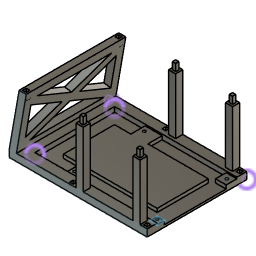
WRO pi EXPANSION BOARD v6 (1) (Autodesk Fusion 360 design; units mm, degrees)
Autodesk Fusion 360 part; units mm, degrees
note: some values were not read from the file. Set by a fixed rule: which sketch regions a step uses.
(part 1 of 2)
sketch "Sketch1" plane through (0, 0, 0) normal (0, 1, 0) x (1, 0, 0)
  line L0 (0, 0) -> (-97, 0)
  line L1 (-97, 0) -> (-97, -5)
  line L2 (-97, -5) -> (0, -5)
  line L3 (0, -5) -> (0, 0)
  dimension "d1" = 97
  dimension "d2" = 5
  constraint horizontal L0
  constraint vertical L1
  constraint horizontal L2
  constraint vertical L3
  constraint coincident L0.start L3.end
  measures "d1" distance of L0.start L0.end
  measures "d2" distance of L0.start L2.end
extrude "Extrude1" add sketch "Sketch1" along normal blind 60
sketch "Sketch2" plane through (0, 0, 5) normal (0, 0, 1) x (-1, 0, 0)
  line L0 (97, 0) -> (0, 0)
  line L1 (0, 0) -> (0, -60)
  line L2 (0, -60) -> (97, -60)
  line L3 (97, -60) -> (97, 0)
  line L4 (0, 0) -> (1.25, 0)
  line L5 (1.25, 0) -> (1.25, -1.25)
  line L6 (1.25, -1.25) -> (3.75, -1.25)
  line L7 (3.75, -1.25) -> (3.75, -3.75)
  line L8 (3.75, -3.75) -> (1.25, -3.75)
  line L9 (1.25, -3.75) -> (1.25, -1.25)
  line L10 (0, -60) -> (0, -58.75)
  line L11 (0, -58.75) -> (1.25, -58.75)
  line L12 (1.25, -58.75) -> (3.75, -58.75)
  line L13 (3.75, -58.75) -> (3.75, -56.25)
  line L14 (3.75, -56.25) -> (1.25, -56.25)
  line L15 (1.25, -56.25) -> (1.25, -58.75)
  line L16 (97, -60) -> (97, -58.75)
  line L17 (97, -58.75) -> (95.75, -58.75)
  line L18 (95.75, -58.75) -> (93.25, -58.75)
  line L19 (93.25, -58.75) -> (93.25, -56.25)
  line L20 (93.25, -56.25) -> (95.75, -56.25)
  line L21 (95.75, -56.25) -> (95.75, -58.75)
  line L22 (97, 0) -> (95.75, 0)
  line L23 (95.75, 0) -> (95.75, -1.25)
  line L24 (95.75, -1.25) -> (93.25, -1.25)
  line L25 (93.25, -1.25) -> (93.25, -3.75)
  line L26 (93.25, -3.75) -> (95.75, -3.75)
  line L27 (95.75, -3.75) -> (95.75, -1.25)
  dimension "d5" = 1.25
  dimension "d6" = 1.25
  dimension "d7" = 2.5
  dimension "d8" = 2.5
  dimension "d9" = 1.25
  dimension "d10" = 1.25
  dimension "d11" = 2.5
  dimension "d12" = 2.5
  dimension "d13" = 1.25
  dimension "d14" = 1.25
  dimension "d15" = 2.5
  dimension "d16" = 2.5
  dimension "d17" = 1.25
  dimension "d18" = 1.25
  dimension "d19" = 2.5
  dimension "d20" = 2.5
  constraint coincident L0.end L1.start
  constraint perpendicular L1 L4
  constraint perpendicular L4 L5
  constraint horizontal L6
  constraint vertical L7
  constraint horizontal L8
  constraint vertical L9
  constraint coincident L1.end L2.start
  constraint perpendicular L2 L10
  constraint perpendicular L10 L11
  constraint horizontal L12
  constraint vertical L13
  constraint horizontal L14
  constraint vertical L15
  constraint coincident L2.end L3.start
  constraint perpendicular L2 L16
  constraint perpendicular L16 L17
  constraint horizontal L18
  constraint vertical L19
  constraint horizontal L20
  constraint vertical L21
  constraint coincident L0.start L3.end
  constraint perpendicular L3 L22
  constraint perpendicular L22 L23
  constraint horizontal L24
  constraint vertical L25
  constraint horizontal L26
  constraint vertical L27
  measures "d5" distance of L0.end L4.end
  measures "d6" distance of L4.end L5.end
  measures "d7" distance of L5.end L6.end
  measures "d8" distance of L5.end L8.end
  measures "d9" distance of L1.end L10.end
  measures "d10" distance of L10.end L11.end
  measures "d11" distance of L11.end L12.end
  measures "d12" distance of L11.end L14.end
  measures "d13" distance of L2.end L16.end
  measures "d14" distance of L16.end L17.end
  measures "d15" distance of L17.end L18.end
  measures "d16" distance of L17.end L20.end
  measures "d17" distance of L0.start L22.end
  measures "d18" distance of L22.end L23.end
  measures "d19" distance of L23.end L24.end
  measures "d20" distance of L23.end L26.end
extrude "Extrude2" cut sketch "Sketch2" against normal blind 1000 contours L6 L7 L8 L9 | L12 L13 L14 L15 | L18 L19 L20 L21 | L24 L25 L26 L27
sketch "Sketch3" plane through (0, 0, 5) normal (0, 0, 1) x (-1, 0, 0)
  line L0 (93.25, -58.75) -> (93.25, -56.25)
  line L1 (93.25, -56.25) -> (95.75, -56.25)
  line L2 (95.75, -56.25) -> (95.75, -58.75)
  line L3 (95.75, -58.75) -> (93.25, -58.75)
  line L4 (3.75, -58.75) -> (1.25, -58.75)
  line L5 (1.25, -58.75) -> (1.25, -56.25)
  line L6 (1.25, -56.25) -> (3.75, -56.25)
  line L7 (3.75, -56.25) -> (3.75, -58.75)
  line L8 (93.25, -1.25) -> (95.75, -1.25)
  line L9 (95.75, -1.25) -> (95.75, -3.75)
  line L10 (95.75, -3.75) -> (93.25, -3.75)
  line L11 (93.25, -3.75) -> (93.25, -1.25)
  line L12 (3.75, -1.25) -> (3.75, -3.75)
  line L13 (3.75, -3.75) -> (1.25, -3.75)
  line L14 (1.25, -3.75) -> (1.25, -1.25)
  line L15 (1.25, -1.25) -> (3.75, -1.25)
  line L16 (97, 0) -> (0, 0)
  line L17 (0, 0) -> (0, -60)
  line L18 (0, -60) -> (97, -60)
  line L19 (97, -60) -> (97, 0)
  line L20 (95.75, -3.75) -> (95.75, -56.25)
  line L21 (95.75, -56.25) -> (95.75, -30)
  line L22 (95.75, -30) -> (95.75, -5)
  line L23 (95.75, -5) -> (95.75, -6.25)
  line L24 (95.75, -6.25) -> (93.25, -6.25)
  line L25 (93.25, -6.25) -> (93.25, -8.75)
  line L26 (93.25, -8.75) -> (95.75, -8.75)
  line L27 (95.75, -8.75) -> (95.75, -6.25)
  line L28 (95.75, -30) -> (95.75, -55)
  line L29 (95.75, -55) -> (95.75, -53.75)
  line L30 (95.75, -53.75) -> (93.25, -53.75)
  line L31 (93.25, -53.75) -> (93.25, -51.25)
  line L32 (93.25, -51.25) -> (95.75, -51.25)
  line L33 (95.75, -51.25) -> (95.75, -53.75)
  line L34 (92, -4) -> (95.75, -4)
  line L35 (95.75, -4) -> (95.75, -0.5684)
  line L36 (95.75, -0.5684) -> (92, -0.5684)
  line L37 (92, -0.5684) -> (92, -4)
  line L38 (93.25, -58.75) -> (96.4667, -58.75)
  line L39 (96.4667, -58.75) -> (96.4667, -55.6639)
  line L40 (96.4667, -55.6639) -> (93.25, -55.6639)
  line L41 (93.25, -55.6639) -> (93.25, -58.75)
  dimension "d23" = 25
  dimension "d24" = 1.25
  dimension "d25" = 2.5
  dimension "d26" = 2.5
  dimension "d27" = 25
  dimension "d28" = 1.25
  dimension "d29" = 2.5
  dimension "d30" = 2.5
  constraint coincident L9.end L10.start
  constraint coincident L1.end L2.start
  constraint midpoint L20 L21.end
  constraint parallel L20 L22
  constraint parallel L20 L23
  constraint horizontal L24
  constraint vertical L25
  constraint horizontal L26
  constraint vertical L27
  constraint parallel L20 L28
  constraint parallel L20 L29
  constraint horizontal L30
  constraint vertical L31
  constraint horizontal L32
  constraint vertical L33
  constraint horizontal L34
  constraint vertical L35
  constraint horizontal L36
  constraint vertical L37
  constraint horizontal L38
  constraint vertical L39
  constraint horizontal L40
  constraint vertical L41
  constraint coincident L0.start L3.end
  measures "d23" distance of L21.end L22.end
  measures "d24" distance of L22.end L23.end
  measures "d25" distance of L23.end L24.end
  measures "d26" distance of L23.end L26.end
  measures "d27" distance of L21.end L28.end
  measures "d28" distance of L28.end L29.end
  measures "d29" distance of L29.end L30.end
  measures "d30" distance of L29.end L32.end
extrude "Extrude3" cut sketch "Sketch3" against normal blind 5 contours L0 L1 L2 L3 L38 L41 | L8 L9 L10 L11 L35 | L20 L22 L24 L25 L26 L27 | L20 L21 L28 L30 L31 L32 L33
sketch "Sketch4" plane through (0, 0, 5) normal (0, 0, 1) x (-1, 0, 0)
  line L0 (93.25, -6.25) -> (95.75, -6.25)
  line L1 (95.75, -6.25) -> (95.75, -8.75)
  line L2 (95.75, -8.75) -> (93.25, -8.75)
  line L3 (93.25, -8.75) -> (93.25, -6.25)
  line L4 (93.25, -53.75) -> (93.25, -51.25)
  line L5 (93.25, -51.25) -> (95.75, -51.25)
  line L6 (95.75, -51.25) -> (95.75, -53.75)
  line L7 (95.75, -53.75) -> (93.25, -53.75)
  line L8 (93.25, -58.75) -> (93.25, -56.25)
  line L9 (93.25, -56.25) -> (95.75, -56.25)
  line L10 (95.75, -56.25) -> (95.75, -58.75)
  line L11 (95.75, -58.75) -> (93.25, -58.75)
  line L12 (3.75, -58.75) -> (1.25, -58.75)
  line L13 (1.25, -58.75) -> (1.25, -56.25)
  line L14 (1.25, -56.25) -> (3.75, -56.25)
  line L15 (3.75, -56.25) -> (3.75, -58.75)
  line L16 (93.25, -1.25) -> (95.75, -1.25)
  line L17 (95.75, -1.25) -> (95.75, -3.75)
  line L18 (95.75, -3.75) -> (93.25, -3.75)
  line L19 (93.25, -3.75) -> (93.25, -1.25)
  line L20 (3.75, -1.25) -> (3.75, -3.75)
  line L21 (3.75, -3.75) -> (1.25, -3.75)
  line L22 (1.25, -3.75) -> (1.25, -1.25)
  line L23 (1.25, -1.25) -> (3.75, -1.25)
  line L24 (97, 0) -> (0, 0)
  line L25 (0, 0) -> (0, -60)
  line L26 (0, -60) -> (97, -60)
  line L27 (97, -60) -> (97, 0)
  line L28 (91.453, -0.7924) -> (95.75, -0.7924)
  line L29 (95.75, -0.7924) -> (95.75, -4.5214)
  line L30 (95.75, -4.5214) -> (91.453, -4.5214)
  line L31 (91.453, -4.5214) -> (91.453, -0.7924)
  line L32 (91.453, -55.7947) -> (95.75, -55.7947)
  line L33 (95.75, -55.7947) -> (95.75, -59.4305)
  line L34 (95.75, -59.4305) -> (91.453, -59.4305)
  line L35 (91.453, -59.4305) -> (91.453, -55.7947)
  constraint horizontal L28
  constraint vertical L29
  constraint horizontal L30
  constraint vertical L31
  constraint horizontal L32
  constraint vertical L33
  constraint horizontal L34
  constraint vertical L35
extrude "Extrude4" add sketch "Sketch4" against normal blind 5 contours L8 L9 L10 L11 L33 | L16 L17 L18 L19 L29
extrude "Extrude5" add 1 faces at (-64.6667, 60, 1.6667) along direction (0, 1, 0) blind 5
extrude "Extrude6" add 1 faces at (-64.6667, 0, 1.6667) along direction (0, -1, 0) blind 5
sketch "Sketch5" plane through (0, 0, 5) normal (0, 0, 1) x (-1, 0, 0)
  line L0 (93.25, -6.25) -> (95.75, -6.25)
  line L1 (95.75, -6.25) -> (95.75, -8.75)
  line L2 (95.75, -8.75) -> (93.25, -8.75)
  line L3 (93.25, -8.75) -> (93.25, -6.25)
  line L4 (93.25, -53.75) -> (93.25, -51.25)
  line L5 (93.25, -51.25) -> (95.75, -51.25)
  line L6 (95.75, -51.25) -> (95.75, -53.75)
  line L7 (95.75, -53.75) -> (93.25, -53.75)
  line L8 (3.75, -58.75) -> (1.25, -58.75)
  line L9 (1.25, -58.75) -> (1.25, -56.25)
  line L10 (1.25, -56.25) -> (3.75, -56.25)
  line L11 (3.75, -56.25) -> (3.75, -58.75)
  line L12 (3.75, -1.25) -> (3.75, -3.75)
  line L13 (3.75, -3.75) -> (1.25, -3.75)
  line L14 (1.25, -3.75) -> (1.25, -1.25)
  line L15 (1.25, -1.25) -> (3.75, -1.25)
  line L16 (0, 5) -> (0, -65)
  line L17 (0, -65) -> (97, -65)
  line L18 (97, -65) -> (97, 5)
  line L19 (97, 5) -> (0, 5)
  line L20 (1.25, -1.25) -> (1.25, 3.75)
  line L21 (1.25, 3.75) -> (3.75, 3.75)
  line L22 (3.75, 3.75) -> (3.75, 1.25)
  line L23 (3.75, 1.25) -> (1.25, 1.25)
  line L24 (1.25, 1.25) -> (1.25, 3.75)
  line L25 (1.25, -58.75) -> (1.25, -63.75)
  line L26 (1.25, -63.75) -> (3.75, -63.75)
  line L27 (3.75, -63.75) -> (3.75, -61.25)
  line L28 (3.75, -61.25) -> (1.25, -61.25)
  line L29 (1.25, -61.25) -> (1.25, -63.75)
  dimension "d39" = 5
  dimension "d40" = 2.5
  dimension "d41" = 2.5
  dimension "d42" = 5
  dimension "d43" = 2.5
  dimension "d44" = 2.5
  constraint coincident L14.end L15.start
  constraint perpendicular L15 L20
  constraint horizontal L21
  constraint vertical L22
  constraint horizontal L23
  constraint vertical L24
  constraint coincident L8.end L9.start
  constraint perpendicular L8 L25
  constraint horizontal L26
  constraint vertical L27
  constraint horizontal L28
  constraint vertical L29
  measures "d39" distance of L14.end L20.end
  measures "d40" distance of L20.end L21.end
  measures "d41" distance of L20.end L23.end
  measures "d42" distance of L8.end L25.end
  measures "d43" distance of L25.end L26.end
  measures "d44" distance of L25.end L28.end
extrude "Extrude7" cut sketch "Sketch5" against normal blind 5000 contours L20 L21 L22 L23 L24 | L25 L26 L27 L28 L29
sketch "Sketch6" plane through (0, 0, 5) normal (0, 0, 1) x (-1, 0, 0)
  line L0 (3.75, 3.75) -> (3.75, 1.25)
  line L1 (3.75, 1.25) -> (1.25, 1.25)
  line L2 (1.25, 1.25) -> (1.25, 3.75)
  line L3 (1.25, 3.75) -> (3.75, 3.75)
  line L4 (3.75, -63.75) -> (1.25, -63.75)
  line L5 (1.25, -63.75) -> (1.25, -61.25)
  line L6 (1.25, -61.25) -> (3.75, -61.25)
  line L7 (3.75, -61.25) -> (3.75, -63.75)
  line L8 (93.25, -6.25) -> (95.75, -6.25)
  line L9 (95.75, -6.25) -> (95.75, -8.75)
  line L10 (95.75, -8.75) -> (93.25, -8.75)
  line L11 (93.25, -8.75) -> (93.25, -6.25)
  line L12 (93.25, -53.75) -> (93.25, -51.25)
  line L13 (93.25, -51.25) -> (95.75, -51.25)
  line L14 (95.75, -51.25) -> (95.75, -53.75)
  line L15 (95.75, -53.75) -> (93.25, -53.75)
  line L16 (3.75, -58.75) -> (1.25, -58.75)
  line L17 (1.25, -58.75) -> (1.25, -56.25)
  line L18 (1.25, -56.25) -> (3.75, -56.25)
  line L19 (3.75, -56.25) -> (3.75, -58.75)
  line L20 (3.75, -1.25) -> (3.75, -3.75)
  line L21 (3.75, -3.75) -> (1.25, -3.75)
  line L22 (1.25, -3.75) -> (1.25, -1.25)
  line L23 (1.25, -1.25) -> (3.75, -1.25)
  line L24 (0, 5) -> (0, -65)
  line L25 (0, -65) -> (97, -65)
  line L26 (97, -65) -> (97, 5)
  line L27 (97, 5) -> (0, 5)
  line L28 (1.25, -58.75) -> (10, -58.75)
  line L29 (10, -58.75) -> (10, 0)
  line L30 (10, 0) -> (1.25, 0)
  line L31 (1.25, 0) -> (1.25, -58.75)
  constraint horizontal L28
  constraint vertical L29
  constraint horizontal L30
  constraint vertical L31
  constraint coincident L16.end L17.start
extrude "Extrude8" add sketch "Sketch6" against normal blind 5 contours L16 L17 L18 L19 L28 L31 | L20 L21 L22 L23 L31
sketch "Sketch7" plane through (0, 0, 5) normal (0, 0, 1) x (-1, 0, 0)
  line L0 (3.75, 3.75) -> (3.75, 1.25)
  line L1 (3.75, 1.25) -> (1.25, 1.25)
  line L2 (1.25, 1.25) -> (1.25, 3.75)
  line L3 (1.25, 3.75) -> (3.75, 3.75)
  line L4 (3.75, -63.75) -> (1.25, -63.75)
  line L5 (1.25, -63.75) -> (1.25, -61.25)
  line L6 (1.25, -61.25) -> (3.75, -61.25)
  line L7 (3.75, -61.25) -> (3.75, -63.75)
  line L8 (93.25, -6.25) -> (95.75, -6.25)
  line L9 (95.75, -6.25) -> (95.75, -8.75)
  line L10 (95.75, -8.75) -> (93.25, -8.75)
  line L11 (93.25, -8.75) -> (93.25, -6.25)
  line L12 (93.25, -53.75) -> (93.25, -51.25)
  line L13 (93.25, -51.25) -> (95.75, -51.25)
  line L14 (95.75, -51.25) -> (95.75, -53.75)
  line L15 (95.75, -53.75) -> (93.25, -53.75)
  line L16 (0, 5) -> (0, -65)
  line L17 (0, -65) -> (97, -65)
  line L18 (97, -65) -> (97, 5)
  line L19 (97, 5) -> (0, 5)
  line L20 (3.75, 3.75) -> (53.25, 3.75)
  line L21 (53.25, 3.75) -> (55.75, 3.75)
  line L22 (55.75, 3.75) -> (55.75, 1.25)
  line L23 (55.75, 1.25) -> (53.25, 1.25)
  line L24 (53.25, 1.25) -> (53.25, 3.75)
  line L25 (3.75, -63.75) -> (53.25, -63.75)
  line L26 (53.25, -63.75) -> (55.75, -63.75)
  line L27 (55.75, -63.75) -> (55.75, -61.25)
  line L28 (55.75, -61.25) -> (53.25, -61.25)
  line L29 (53.25, -61.25) -> (53.25, -63.75)
  dimension "d49" = 49.5
  dimension "d50" = 2.5
  dimension "d51" = 2.5
  dimension "d52" = 49.5
  dimension "d53" = 2.5
  dimension "d54" = 2.5
  constraint coincident L0.start L3.end
  constraint perpendicular L0 L20
  constraint horizontal L21
  constraint vertical L22
  constraint horizontal L23
  constraint vertical L24
  constraint coincident L4.start L7.end
  constraint perpendicular L7 L25
  constraint horizontal L26
  constraint vertical L27
  constraint horizontal L28
  constraint vertical L29
  measures "d49" distance of L0.start L20.end
  measures "d50" distance of L20.end L21.end
  measures "d51" distance of L20.end L23.end
  measures "d52" distance of L4.start L25.end
  measures "d53" distance of L25.end L26.end
  measures "d54" distance of L25.end L28.end
extrude "Extrude9" cut sketch "Sketch7" against normal blind 150 contours L21 L22 L23 L24 | L26 L27 L28 L29
sketch "Sketch8" plane through (0, 0, 5) normal (0, 0, 1) x (-1, 0, 0)
  line L0 (55.75, 3.75) -> (55.75, 1.25)
  line L1 (55.75, 1.25) -> (53.25, 1.25)
  line L2 (53.25, 1.25) -> (53.25, 3.75)
  line L3 (53.25, 3.75) -> (55.75, 3.75)
  line L4 (55.75, -63.75) -> (53.25, -63.75)
  line L5 (53.25, -63.75) -> (53.25, -61.25)
  line L6 (53.25, -61.25) -> (55.75, -61.25)
  line L7 (55.75, -61.25) -> (55.75, -63.75)
  line L8 (3.75, 3.75) -> (3.75, 1.25)
  line L9 (3.75, 1.25) -> (1.25, 1.25)
  line L10 (1.25, 1.25) -> (1.25, 3.75)
  line L11 (1.25, 3.75) -> (3.75, 3.75)
  line L12 (3.75, -63.75) -> (1.25, -63.75)
  line L13 (1.25, -63.75) -> (1.25, -61.25)
  line L14 (1.25, -61.25) -> (3.75, -61.25)
  line L15 (3.75, -61.25) -> (3.75, -63.75)
  line L16 (93.25, -6.25) -> (95.75, -6.25)
  line L17 (95.75, -6.25) -> (95.75, -8.75)
  line L18 (95.75, -8.75) -> (93.25, -8.75)
  line L19 (93.25, -8.75) -> (93.25, -6.25)
  line L20 (93.25, -53.75) -> (93.25, -51.25)
  line L21 (93.25, -51.25) -> (95.75, -51.25)
  line L22 (95.75, -51.25) -> (95.75, -53.75)
  line L23 (95.75, -53.75) -> (93.25, -53.75)
  line L24 (0, 5) -> (0, -65)
  line L25 (0, -65) -> (97, -65)
  line L26 (97, -65) -> (97, 5)
  line L27 (97, 5) -> (0, 5)
  line L28 (86.4798, -65) -> (86.4798, -30)
  line L29 (86.4798, -30) -> (86.4798, -2)
  line L30 (86.4798, -2) -> (0.4798, -2)
  line L31 (0.4798, -2) -> (0.4798, -58)
  line L32 (0.4798, -58) -> (86.4798, -58)
  line L33 (86.4798, -58) -> (86.4798, -2)
  dimension "d57" = 35
  dimension "d58" = 28
  dimension "d59" = 86
  dimension "d60" = 56
  constraint coincident L25 L28.start
  constraint perpendicular L27 L28
  constraint perpendicular L25 L29
  constraint horizontal L30
  constraint vertical L31
  constraint horizontal L32
  constraint vertical L33
  measures "d57" distance of L28.start L28.end
  measures "d58" distance of L28.end L29.end
  measures "d59" distance of L29.end L30.end
  measures "d60" distance of L29.end L32.end
extrude "Extrude10" cut sketch "Sketch8" against normal blind 1 contours L28 L29 L30 L31 L32 L33
sketch "Sketch9" plane through (0, 0, 5) normal (0, 0, 1) x (-1, 0, 0)
  line L0 (0.4798, -2) -> (86.4798, -2)
  line L1 (86.4798, -2) -> (86.4798, -58)
  line L2 (86.4798, -58) -> (0.4798, -58)
  line L3 (0.4798, -58) -> (0.4798, -2)
  line L4 (55.75, 3.75) -> (55.75, 1.25)
  line L5 (55.75, 1.25) -> (53.25, 1.25)
  line L6 (53.25, 1.25) -> (53.25, 3.75)
  line L7 (53.25, 3.75) -> (55.75, 3.75)
  line L8 (55.75, -63.75) -> (53.25, -63.75)
  line L9 (53.25, -63.75) -> (53.25, -61.25)
  line L10 (53.25, -61.25) -> (55.75, -61.25)
  line L11 (55.75, -61.25) -> (55.75, -63.75)
  line L12 (3.75, 3.75) -> (3.75, 1.25)
  line L13 (3.75, 1.25) -> (1.25, 1.25)
  line L14 (1.25, 1.25) -> (1.25, 3.75)
  line L15 (1.25, 3.75) -> (3.75, 3.75)
  line L16 (3.75, -63.75) -> (1.25, -63.75)
  line L17 (1.25, -63.75) -> (1.25, -61.25)
  line L18 (1.25, -61.25) -> (3.75, -61.25)
  line L19 (3.75, -61.25) -> (3.75, -63.75)
  line L20 (93.25, -6.25) -> (95.75, -6.25)
  line L21 (95.75, -6.25) -> (95.75, -8.75)
  line L22 (95.75, -8.75) -> (93.25, -8.75)
  line L23 (93.25, -8.75) -> (93.25, -6.25)
  line L24 (93.25, -53.75) -> (93.25, -51.25)
  line L25 (93.25, -51.25) -> (95.75, -51.25)
  line L26 (95.75, -51.25) -> (95.75, -53.75)
  line L27 (95.75, -53.75) -> (93.25, -53.75)
  line L28 (0, 5) -> (0, -65)
  line L29 (0, -65) -> (97, -65)
  line L30 (97, -65) -> (97, 5)
  line L31 (97, 5) -> (0, 5)
  line L32 (86.4798, -2) -> (85.9998, -2)
  line L33 (85.9998, -2) -> (85.9998, -59.3993)
  line L34 (85.9998, -59.3993) -> (86.4798, -59.3993)
  line L35 (86.4798, -59.3993) -> (86.4798, -2)
  dimension "d63" = 0.48
  constraint horizontal L32
  constraint vertical L33
  constraint horizontal L34
  constraint vertical L35
  constraint coincident L0.end L1.start
  measures "d63" distance of L0.end L32.end
extrude "Extrude11" add sketch "Sketch9" against normal blind 2 contours L0 L1 L2 L32 L33 L35
sketch "Sketch10" plane through (0, 0, 5) normal (0, 0, 1) x (-1, 0, 0)
  line L0 (0.4798, -2) -> (85.9998, -2)
  line L1 (85.9998, -2) -> (85.9998, -58)
  line L2 (85.9998, -58) -> (0.4798, -58)
  line L3 (0.4798, -58) -> (0.4798, -2)
  line L4 (55.75, 3.75) -> (55.75, 1.25)
  line L5 (55.75, 1.25) -> (53.25, 1.25)
  line L6 (53.25, 1.25) -> (53.25, 3.75)
  line L7 (53.25, 3.75) -> (55.75, 3.75)
  line L8 (55.75, -63.75) -> (53.25, -63.75)
  line L9 (53.25, -63.75) -> (53.25, -61.25)
  line L10 (53.25, -61.25) -> (55.75, -61.25)
  line L11 (55.75, -61.25) -> (55.75, -63.75)
  line L12 (3.75, 3.75) -> (3.75, 1.25)
  line L13 (3.75, 1.25) -> (1.25, 1.25)
  line L14 (1.25, 1.25) -> (1.25, 3.75)
  line L15 (1.25, 3.75) -> (3.75, 3.75)
  line L16 (3.75, -63.75) -> (1.25, -63.75)
  line L17 (1.25, -63.75) -> (1.25, -61.25)
  line L18 (1.25, -61.25) -> (3.75, -61.25)
  line L19 (3.75, -61.25) -> (3.75, -63.75)
  line L20 (93.25, -6.25) -> (95.75, -6.25)
  line L21 (95.75, -6.25) -> (95.75, -8.75)
  line L22 (95.75, -8.75) -> (93.25, -8.75)
  line L23 (93.25, -8.75) -> (93.25, -6.25)
  line L24 (93.25, -53.75) -> (93.25, -51.25)
  line L25 (93.25, -51.25) -> (95.75, -51.25)
  line L26 (95.75, -51.25) -> (95.75, -53.75)
  line L27 (95.75, -53.75) -> (93.25, -53.75)
  line L28 (0, 5) -> (0, -65)
  line L29 (0, -65) -> (97, -65)
  line L30 (97, -65) -> (97, 5)
  line L31 (97, 5) -> (0, 5)
  line L32 (0.4798, -58) -> (-1.0163, -58)
  line L33 (-1.0163, -58) -> (-1.0163, -2)
  line L34 (-1.0163, -2) -> (0.4798, -2)
  line L35 (0.4798, -2) -> (0.4798, -58)
  constraint horizontal L32
  constraint vertical L33
  constraint horizontal L34
  constraint vertical L35
  constraint coincident L2.end L3.start
extrude "Extrude12" cut sketch "Sketch10" against normal blind 1 contours L3 L28 L32 L34 L35
sketch "Sketch11" plane through (0, 0, 4) normal (0, 0, 1) x (-1, 0, 0)
  line L0 (85.9998, -58) -> (85.9998, -2)
  line L1 (85.9998, -2) -> (0, -2)
  line L2 (0, -2) -> (0, -58)
  line L3 (0, -58) -> (85.9998, -58)
  line L4 (0, -58) -> (2.5, -58)
  line L5 (2.5, -58) -> (2.5, -55.5)
  line L6 (2.5, -55.5) -> (3.5, -55.5)
  line L7 (3.5, -55.5) -> (3.5, -54.5)
  circle A0 centre (3.5, -54.5) radius 1
  line L8 (0, -2) -> (3.5, -2)
  line L9 (3.5, -2) -> (3.5, -5.5)
  circle A1 centre (3.5, -5.5) radius 1
  dimension "d68" = 2.5
  dimension "d69" = 2.5
  dimension "d70" = 1
  dimension "d71" = 1
  dimension "d72" = 2
  dimension "d73" = 3.5
  dimension "d74" = 3.5
  dimension "d75" = 2
  constraint coincident L2.end L3.start
  constraint perpendicular L2 L4
  constraint perpendicular L4 L5
  constraint perpendicular L5 L6
  constraint perpendicular L6 L7
  constraint coincident L7.end A0.centre
  constraint coincident L1.end L2.start
  constraint perpendicular L2 L8
  constraint perpendicular L8 L9
  constraint coincident L9.end A1.centre
  measures "d68" distance of L2.end L4.end
  measures "d69" distance of L4.end L5.end
  measures "d70" distance of L5.end L6.end
  measures "d71" distance of L6.end L7.end
  measures "d72" diameter of A0
  measures "d73" distance of L1.end L8.end
  measures "d74" distance of L8.end L9.end
  measures "d75" diameter of A1
extrude "Extrude13" cut sketch "Sketch11" against normal blind 100 contours A0 | A1
sketch "Sketch12" plane through (0, 0, 4) normal (0, 0, 1) x (-1, 0, 0)
  circle A0 centre (3.5, -5.5) radius 1
  circle A1 centre (3.5, -54.5) radius 1
  line L0 (85.9998, -58) -> (85.9998, -2)
  line L1 (5, -7) -> (0, -7)
  line L2 (0, -7) -> (0, -2)
  line L3 (0, -2) -> (5, -2)
  line L4 (5, -2) -> (5, -7)
  constraint horizontal L1
  constraint vertical L2
  constraint horizontal L3
  constraint vertical L4
sketch "Sketch13" plane through (0, 0, 4) normal (0, 0, 1) x (-1, 0, 0)
sketch "Sketch14" plane through (0, 0, 4) normal (0, 0, 1) x (-1, 0, 0)
  line L0 (0, -58) -> (3.5, -58)
  line L1 (3.5, -58) -> (3.5, -54.5)
  line L2 (3.5, -54.5) -> (61.5, -54.5)
  circle A0 centre (61.5, -54.5) radius 1
  line L3 (61.5, -54.5) -> (61.5, -5.5)
  circle A1 centre (61.5, -5.5) radius 1
  dimension "d82" = 3.5
  dimension "d83" = 3.5
  dimension "d84" = 58
  dimension "d85" = 2
  dimension "d86" = 49
  dimension "d87" = 2
  constraint horizontal L0
  constraint perpendicular L0 L1
  constraint perpendicular L1 L2
  constraint coincident L2.end A0.centre
  constraint perpendicular L2 L3
  constraint coincident L3.end A1.centre
  measures "d82" distance of L0.start L0.end
  measures "d83" distance of L0.end L1.end
  measures "d84" distance of L1.end L2.end
  measures "d85" diameter of A0
  measures "d86" distance of L2.end L3.end
  measures "d87" diameter of A1
extrude "Extrude14" cut sketch "Sketch14" against normal blind 500
sketch "Sketch15" plane through (0, 0, 4) normal (0, 0, 1) x (-1, 0, 0)
  circle A0 centre (61.5, -54.5) radius 1
  circle A1 centre (61.5, -5.5) radius 1
  circle A2 centre (3.5, -5.5) radius 1
  circle A3 centre (3.5, -54.5) radius 1
  line L0 (85.9998, -58) -> (85.9998, -2)
  line L1 (85.9998, -2) -> (0, -2)
  line L2 (0, -2) -> (0, -58)
  line L3 (0, -58) -> (85.9998, -58)
  line L4 (0, -58) -> (0, -2)
  line L5 (64.5, -58) -> (52.5, -58)
  line L6 (52.5, -58) -> (52.5, -51)
  line L7 (64.5, -51) -> (64.5, -58)
  line L8 (60.5, -5.5) -> (57.5, -5.5)
  line L9 (62.5, -5.5) -> (64, -5.5)
  line L10 (57.5, -5.5) -> (57.5, -2)
  line L11 (57.5, -2) -> (64, -2)
  line L12 (64, -2) -> (64, -9)
  line L13 (57.5, -9) -> (57.5, -2)
  line L14 (64.5, -58) -> (52.5, -58)
  line L15 (52.5, -58) -> (52.5, -48)
  line L16 (52.5, -48) -> (64.5, -48)
  line L17 (64.5, -48) -> (64.5, -58)
  line L18 (57.5, -2) -> (64, -2)
  line L19 (64, -2) -> (64, -12)
  line L20 (64, -12) -> (57.5, -12)
  line L21 (57.5, -12) -> (57.5, -2)
  line L22 (0, -43) -> (10, -43)
  line L23 (10, -43) -> (10, -58)
  line L24 (52.5, -48) -> (10, -48)
  line L25 (64, -12) -> (76, -12)
  line L26 (76, -12) -> (10, -12)
  line L27 (10, -12) -> (10, -48)
  line L28 (10, -48) -> (76, -48)
  line L29 (76, -48) -> (76, -12)
  dimension "d92" = 7
  dimension "d93" = 3
  dimension "d94" = 1.5
  dimension "d95" = 7
  dimension "d96" = 10
  dimension "d97" = 10
  dimension "d98" = 10
  dimension "d99" = 12
  constraint coincident L2.end L3.start
  constraint coincident L1.end L2.start
  constraint horizontal L5
  constraint vertical L6
  constraint vertical L7
  constraint coincident L3 L5.start
  constraint coincident A1 L8.start
  constraint parallel L1 L8
  constraint coincident A1 L9.start
  constraint parallel L1 L9
  constraint coincident L1 L10.end
  constraint perpendicular L1 L10
  constraint horizontal L11
  constraint vertical L12
  constraint vertical L13
  constraint horizontal L14
  constraint vertical L15
  constraint horizontal L16
  constraint vertical L17
  constraint horizontal L18
  constraint vertical L19
  constraint horizontal L20
  constraint vertical L21
  constraint coincident L4 L22.start
  constraint perpendicular L4 L22
  constraint coincident L3 L23.end
  constraint perpendicular L3 L23
  constraint coincident L23 L24.end
  constraint perpendicular L23 L24
  constraint perpendicular L0 L25
  constraint horizontal L26
  constraint vertical L27
  constraint horizontal L28
  constraint vertical L29
  measures "d92" distance of L5.start L7.start
  measures "d93" distance of L8.start L8.end
  measures "d94" distance of L9.start L9.end
  measures "d95" distance of L10.end L13.start
  measures "d96" distance of L5.start L16.end
  measures "d97" distance of L10.end L20.end
  measures "d98" distance of L22.start L22.end
  measures "d99" distance of L19.end L25.end
extrude "Extrude15" cut sketch "Sketch15" against normal blind 2.5 contours L0 L1 L3 L7 L12 L17 L19 L25 L26 L28 L29 | L3 L6 L15 L23 L24 L28
sketch "Sketch16" plane through (0, 0, 4) normal (0, 0, 1) x (-1, 0, 0)
  circle A0 centre (3.5, -54.5) radius 1
  circle A1 centre (3.5, -5.5) radius 1
  circle A2 centre (61.5, -5.5) radius 1
  circle A3 centre (61.5, -54.5) radius 1
  line L0 (10, -58) -> (10, -48)
  line L1 (10, -48) -> (52.5, -48)
  line L2 (52.5, -48) -> (52.5, -58)
  line L3 (52.5, -58) -> (64.5, -58)
  line L4 (64.5, -58) -> (64.5, -48)
  line L5 (64.5, -48) -> (76, -48)
  line L6 (76, -48) -> (76, -12)
  line L7 (76, -12) -> (64, -12)
  line L8 (64, -12) -> (64, -2)
  line L9 (64, -2) -> (0, -2)
  line L10 (0, -2) -> (0, -58)
  line L11 (0, -58) -> (10, -58)
  line L12 (0, -58) -> (7.5, -58)
  line L13 (7.5, -58) -> (7.5, -50.5)
  line L14 (7.5, -50.5) -> (0, -50.5)
  line L15 (0, -50.5) -> (0, -58)
  line L16 (0, -2) -> (5, -2)
  line L17 (5, -2) -> (5, -7)
  line L18 (5, -7) -> (0, -7)
  line L19 (0, -7) -> (0, -2)
  line L20 (10, -48) -> (76, -48)
  line L21 (76, -48) -> (76, -12)
  line L22 (76, -12) -> (10, -12)
  line L23 (10, -12) -> (10, -48)
  line L24 (64, -2) -> (57.5, -2)
  line L25 (57.5, -2) -> (57.5, -13.1348)
  line L26 (57.5, -13.1348) -> (64, -13.1348)
  line L27 (64, -13.1348) -> (64, -2)
  dimension "d102" = 7.5
  dimension "d103" = 7.5
  dimension "d104" = 6.5
  constraint horizontal L12
  constraint vertical L13
  constraint horizontal L14
  constraint vertical L15
  constraint coincident L10.end L11.start
  constraint horizontal L16
  constraint vertical L17
  constraint horizontal L18
  constraint vertical L19
  constraint coincident L9.end L10.start
  constraint horizontal L20
  constraint vertical L21
  constraint horizontal L22
  constraint vertical L23
  constraint coincident L6.end L7.start
  constraint coincident L0.end L1.start
  constraint horizontal L24
  constraint vertical L25
  constraint horizontal L26
  constraint vertical L27
  constraint coincident L8.end L9.start
  measures "d102" distance of L10.end L12.end
  measures "d103" distance of L10.end L14.end
  measures "d104" distance of L8.end L24.end
extrude "Extrude16" cut sketch "Sketch16" against normal blind 2.5 contours L0 L9 L10 L11 L13 L14 L17 L18 L22 L23 L25
sketch "Sketch17" plane through (0, -5, 0) normal (0, -1, 0) x (1, 0, 0)
  line L0 (0, 0) -> (0, 5)
  line L1 (0, 5) -> (-97, 5)
  line L2 (-97, 5) -> (-97, 0)
  line L3 (-97, 0) -> (0, 0)
  line L4 (-97, 5) -> (-90.0541, 44.3923)
  line L5 (-97, 5) -> (-57, 5) construction
  line L6 (-92.3722, 31.2455) -> (-87.6738, 29.5354)
  line L7 (-92.3722, 31.2455) -> (-87.3722, 31.2455) construction
  line L8 (-94.8047, 17.45) -> (-90.1063, 15.7399)
  line L9 (-94.8047, 17.45) -> (-89.8047, 17.45) construction
  line L10 (-87.6738, 29.5354) -> (-92, 5)
  line L11 (-87.6738, 29.5354) -> (-62.7599, 29.5354) construction
  line L12 (-92, 5) -> (-85.0541, 44.3923)
  line L13 (-90.0541, 44.3923) -> (-85.0541, 44.3923)
  dimension "d107" = 80
  dimension "d108" = 40
  dimension "d109" = 20
  dimension "d110" = 5
  dimension "d111" = 20
  dimension "d112" = 5
  dimension "d113" = 100
  dimension "d114" = 40
  constraint horizontal L5
  constraint coincident L1.end L2.start
  constraint horizontal L7
  constraint coincident L4 L6.start
  constraint horizontal L9
  constraint coincident L4 L8.start
  constraint horizontal L11
  constraint coincident L5 L10.end
  constraint parallel L10 L12
  measures "d107" angle of L4 L5
  measures "d108" distance of L1.end L4.end
  measures "d109" angle of L6 L7
  measures "d110" distance of L6.start L6.end
  measures "d111" angle of L8 L9
  measures "d112" distance of L8.start L8.end
  measures "d113" angle of L10 L11
  measures "d114" distance of L10.end L12.end
extrude "Extrude17" add sketch "Sketch17" against normal blind 70 contours L1 L4 L8 L10 L12 | L4 L6 L8 L10 L12 | L4 L6 L12 L13
sketch "Sketch18" plane through (0, -5, 0) normal (0, -1, 0) x (1, 0, 0)
  line L0 (0, 0) -> (0, 5)
  line L1 (0, 5) -> (-92, 5)
  line L2 (-92, 5) -> (-85.0541, 44.3923)
  line L3 (-85.0541, 44.3923) -> (-90.0541, 44.3923)
  line L4 (-90.0541, 44.3923) -> (-97, 5)
  line L5 (-97, 5) -> (-97, 0)
  line L6 (-97, 0) -> (0, 0)
sketch "Sketch19" plane through (0, 0, 44.3923) normal (0, 0, 1) x (-1, 0, 0)
  line L0 (90.0541, 5) -> (85.0541, 5)
  line L1 (85.0541, 5) -> (85.0541, -65)
  line L2 (85.0541, -65) -> (90.0541, -65)
  line L3 (90.0541, -65) -> (90.0541, 5)
  line L4 (90.0541, 5) -> (90.0541, 3.65)
  line L5 (90.0541, 3.65) -> (88.7041, 3.65)
  line L6 (88.7041, 3.65) -> (86.4041, 3.65)
  line L7 (86.4041, 3.65) -> (86.4041, 1.35)
  line L8 (86.4041, 1.35) -> (88.7041, 1.35)
  line L9 (88.7041, 1.35) -> (88.7041, 3.65)
  dimension "d117" = 1.35
  dimension "d118" = 1.35
  dimension "d119" = 2.3
  dimension "d120" = 2.3
  constraint coincident L0.start L3.end
  constraint perpendicular L0 L4
  constraint perpendicular L4 L5
  constraint horizontal L6
  constraint vertical L7
  constraint horizontal L8
  constraint vertical L9
  measures "d117" distance of L0.start L4.end
  measures "d118" distance of L4.end L5.end
  measures "d119" distance of L5.end L6.end
  measures "d120" distance of L5.end L8.end
extrude "Extrude18" add sketch "Sketch19" along normal blind 5 contours L6 L7 L8 L9
sketch "Sketch20" plane through (0, 0, 44.3923) normal (0, 0, 1) x (-1, 0, 0)
  line L0 (88.7041, 1.35) -> (86.4041, 1.35)
  line L1 (86.4041, 1.35) -> (86.4041, 3.65)
  line L2 (86.4041, 3.65) -> (88.7041, 3.65)
  line L3 (88.7041, 3.65) -> (88.7041, 1.35)
  line L4 (90.0541, 5) -> (85.0541, 5)
  line L5 (85.0541, 5) -> (85.0541, -65)
  line L6 (85.0541, -65) -> (90.0541, -65)
  line L7 (90.0541, -65) -> (90.0541, 5)
  line L8 (90.0541, -65) -> (88.8041, -65)
  line L9 (88.8041, -65) -> (88.8041, -63.75)
  line L10 (88.8041, -63.75) -> (90.0541, -63.75)
  line L11 (90.0541, -63.75) -> (90.0541, -65)
  line L12 (88.8041, -63.75) -> (86.5041, -63.75)
  line L13 (86.5041, -63.75) -> (86.5041, -61.45)
  line L14 (86.5041, -61.45) -> (88.8041, -61.45)
  line L15 (88.8041, -61.45) -> (88.8041, -63.75)
  dimension "d123" = 1.25
  dimension "d124" = 1.25
  dimension "d125" = 2.3
  dimension "d126" = 2.3
  constraint horizontal L8
  constraint vertical L9
  constraint horizontal L10
  constraint vertical L11
  constraint coincident L6.end L7.start
  constraint horizontal L12
  constraint vertical L13
  constraint horizontal L14
  constraint vertical L15
  measures "d123" distance of L6.end L8.end
  measures "d124" distance of L6.end L10.end
  measures "d125" distance of L9.end L12.end
  measures "d126" distance of L9.end L14.end
extrude "Extrude19" add sketch "Sketch20" along normal blind 5 contours L12 L13 L14 L15
extrude "Extrude20" cut 2 faces at (-87.1707, -2.8833, 49.3923) (-88.0374, 62.9833, 49.3923) along direction (0, 0, -1) blind 10
sketch "Sketch21" plane through (-94.9301, 0, 16.7387) normal (-0.984808, 0, 0.173648) x (0, -1, 0)
  line L0 (5, -11.9198) -> (5, 28.0802)
  line L1 (5, 28.0802) -> (-65, 28.0802)
  line L2 (-65, 28.0802) -> (-65, -11.9198)
  line L3 (-65, -11.9198) -> (5, -11.9198)
  line L4 (-58.8433, 28.0802) -> (-58.8433, 23.0802)
  line L5 (-65, 23) -> (-60, 23)
  line L6 (-60, 23) -> (0, 23)
  line L7 (0, 23) -> (0, -7)
  line L8 (0, -7) -> (-60, -7)
  line L9 (-60, -7) -> (-60, 23)
  line L10 (-60, -7) -> (-56, -7)
  line L11 (-60, -7) -> (-60, -3)
  line L12 (0, 23) -> (0, 19)
  line L13 (0, 23) -> (0, 19)
  line L14 (0, 23) -> (-4, 23)
  line L15 (-60, 23) -> (-60, 19)
  line L16 (-60, 23) -> (-56, 23)
  line L17 (0, -7) -> (0, -3)
  line L18 (0, -7) -> (-4, -7)
  line L19 (-56, 23) -> (0, -3)
  line L20 (-4, -7) -> (-60, 19)
  line L21 (-56, -7) -> (0, 19)
  line L22 (-4, 23) -> (-60, -3)
  dimension "d131" = 5
  dimension "d132" = 5
  dimension "d133" = 60
  dimension "d134" = 30
  dimension "d135" = 4
  dimension "d136" = 4
  dimension "d137" = 4
  dimension "d138" = 4
  dimension "d139" = 4
  dimension "d140" = 4
  dimension "d141" = 4
  dimension "d142" = 4
  constraint coincident L1 L4.start
  constraint perpendicular L1 L4
  constraint coincident L2 L5.start
  constraint perpendicular L2 L5
  constraint horizontal L6
  constraint vertical L7
  constraint horizontal L8
  constraint vertical L9
  constraint perpendicular L9 L10
  constraint perpendicular L8 L11
  constraint coincident L7 L12.end
  constraint perpendicular L6 L13
  constraint perpendicular L7 L14
  constraint perpendicular L6 L15
  constraint perpendicular L4 L16
  constraint perpendicular L8 L17
  constraint perpendicular L7 L18
  measures "d131" distance of L4.start L4.end
  measures "d132" distance of L5.start L5.end
  measures "d133" distance of L5.end L6.end
  measures "d134" distance of L5.end L8.end
  measures "d135" distance of L8.end L10.end
  measures "d136" distance of L8.end L11.end
  measures "d137" distance of L6.end L12.end
  measures "d138" distance of L6.end L14.end
  measures "d139" distance of L5.end L15.end
  measures "d140" distance of L5.end L16.end
  measures "d141" distance of L7.end L17.end
  measures "d142" distance of L7.end L18.end
extrude "Extrude21" cut sketch "Sketch21" against normal blind 5 contours L6 L19 L22 | L9 L20 L22 | L7 L19 L21 | L8 L20 L21
sketch "Sketch22" plane through (0, 65, 0) normal (0, 1, 0) x (-1, 0, 0)
  line L0 (0, 5) -> (0, 0)
  line L1 (97, 0) -> (97, 5)
  line L2 (97, 5) -> (90.0541, 44.3923)
  line L3 (90.0541, 44.3923) -> (85.0541, 44.3923)
  line L4 (85.0541, 44.3923) -> (92, 5)
  line L5 (92, 5) -> (0, 5)
sketch "Sketch23" plane through (0, 0, 44.3923) normal (0, 0, 1) x (-1, 0, 0)
  line L0 (88.8041, -61.45) -> (88.8041, -63.75)
  line L1 (88.8041, -63.75) -> (86.5041, -63.75)
  line L2 (86.5041, -63.75) -> (86.5041, -61.45)
  line L3 (86.5041, -61.45) -> (88.8041, -61.45)
  line L4 (88.7041, 1.35) -> (86.4041, 1.35)
  line L5 (86.4041, 1.35) -> (86.4041, 3.65)
  line L6 (86.4041, 3.65) -> (88.7041, 3.65)
  line L7 (88.7041, 3.65) -> (88.7041, 1.35)
  line L8 (90.0541, 5) -> (85.0541, 5)
  line L9 (85.0541, 5) -> (85.0541, -65)
  line L10 (85.0541, -65) -> (90.0541, -65)
  line L11 (90.0541, -65) -> (90.0541, 5)
  line L12 (88.7041, 1.35) -> (88.7041, 1.25)
  line L13 (88.7041, 1.35) -> (88.8041, 1.35)
  line L14 (88.8039, 1.25) -> (86.3039, 1.25)
  line L15 (86.3039, 1.25) -> (86.3039, 3.75)
  line L16 (86.3039, 3.75) -> (88.8039, 3.75)
  line L17 (88.8039, 3.75) -> (88.8039, 1.25)
  line L18 (88.8041, -63.75) -> (88.9041, -63.75)
  line L19 (88.9041, -63.75) -> (88.9041, -63.85)
  line L20 (88.9041, -63.85) -> (86.4041, -63.85)
  line L21 (86.4041, -63.85) -> (86.4041, -61.35)
  line L22 (86.4041, -61.35) -> (88.9041, -61.35)
  line L23 (88.9041, -61.35) -> (88.9041, -63.85)
  dimension "d145" = 0.1
  dimension "d146" = 0.1
  dimension "d147" = 2.5
  dimension "d148" = 2.5
  dimension "d149" = 0.1
  dimension "d150" = 0.1
  dimension "d151" = 2.5
  dimension "d152" = 2.5
  constraint coincident L4.start L7.end
  constraint vertical L12
  constraint perpendicular L7 L13
  constraint horizontal L14
  constraint vertical L15
  constraint horizontal L16
  constraint vertical L17
  constraint coincident L0.end L1.start
  constraint perpendicular L0 L18
  constraint perpendicular L18 L19
  constraint horizontal L20
  constraint vertical L21
  constraint horizontal L22
  constraint vertical L23
  measures "d145" distance of L4.start L12.end
  measures "d146" distance of L4.start L13.end
  measures "d147" distance of L14.start L14.end
  measures "d148" distance of L14.start L16.end
  measures "d149" distance of L0.end L18.end
  measures "d150" distance of L18.end L19.end
  measures "d151" distance of L19.end L20.end
  measures "d152" distance of L19.end L22.end
extrude "Extrude22" cut sketch "Sketch23" against normal blind 5 contours L12 L13 L14 L15 L16 L17 | L19 L20 L21 L22 L23
sketch "Sketch24" plane through (0, -5, 0) normal (0, -1, 0) x (1, 0, 0)
sketch "Sketch25" plane through (0, 0, 5) normal (0, 0, 1) x (-1, 0, 0)
  line L0 (92, -65) -> (92, 5)
  line L1 (92, 5) -> (0, 5)
  line L2 (0, 5) -> (0, -2)
  line L3 (0, -2) -> (85.9998, -2)
  line L4 (85.9998, -2) -> (85.9998, -58)
  line L5 (85.9998, -58) -> (0, -58)
  line L6 (0, -58) -> (0, -65)
  line L7 (0, -65) -> (92, -65)
  line L8 (55.75, 3.75) -> (55.75, 1.25)
  line L9 (55.75, 1.25) -> (53.25, 1.25)
  line L10 (53.25, 1.25) -> (53.25, 3.75)
  line L11 (53.25, 3.75) -> (55.75, 3.75)
  line L12 (55.75, -63.75) -> (53.25, -63.75)
  line L13 (53.25, -63.75) -> (53.25, -61.25)
  line L14 (53.25, -61.25) -> (55.75, -61.25)
  line L15 (55.75, -61.25) -> (55.75, -63.75)
  line L16 (3.75, 3.75) -> (3.75, 1.25)
  line L17 (3.75, 1.25) -> (1.25, 1.25)
  line L18 (1.25, 1.25) -> (1.25, 3.75)
  line L19 (1.25, 3.75) -> (3.75, 3.75)
  line L20 (3.75, -63.75) -> (1.25, -63.75)
  line L21 (1.25, -63.75) -> (1.25, -61.25)
  line L22 (1.25, -61.25) -> (3.75, -61.25)
  line L23 (3.75, -61.25) -> (3.75, -63.75)
  line L24 (50, 5) -> (50, 3.65)
  line L25 (50, 3.65) -> (48.65, 3.65)
  line L26 (48.65, 3.65) -> (46.35, 3.65)
  line L27 (46.35, 3.65) -> (46.35, 1.35)
  line L28 (46.35, 1.35) -> (48.65, 1.35)
  line L29 (48.65, 1.35) -> (48.65, 3.65)
  dimension "d159" = 1.35
  dimension "d160" = 1.35
  dimension "d161" = 2.3
  dimension "d162" = 2.3
  constraint coincident L1 L24.start
  constraint perpendicular L1 L24
  constraint perpendicular L24 L25
  constraint horizontal L26
  constraint vertical L27
  constraint horizontal L28
  constraint vertical L29
  measures "d159" distance of L24.start L24.end
  measures "d160" distance of L24.end L25.end
  measures "d161" distance of L25.end L26.end
  measures "d162" distance of L25.end L28.end
extrude "Extrude23" add sketch "Sketch25" along normal blind 50 contours L26 L27 L28 L29
sketch "Sketch26" plane through (0, -5, 0) normal (0, -1, 0) x (1, 0, 0)
  line L0 (-92, 5) -> (-85.0541, 44.3923)
  line L1 (-92, 5) -> (-52, 5) construction
  line L2 (-85.0541, 44.3923) -> (-46, 44.3923)
  line L3 (-46, 44.3923) -> (-46, 49.3923)
  line L4 (-46, 44.3923) -> (-49.5907, 44.3923)
  line L5 (-49.5907, 44.3923) -> (-49.5907, 49.3923)
  line L6 (-49.5907, 49.3923) -> (-46, 49.3923)
  line L7 (-46, 49.3923) -> (-46, 44.3923)
  line L8 (-46, 49.3923) -> (-51.6958, 49.3923)
  line L9 (-51.6958, 49.3923) -> (-51.6958, 56.6847)
  line L10 (-51.6958, 56.6847) -> (-46, 56.6847)
  line L11 (-46, 56.6847) -> (-46, 49.3923)
  dimension "d165" = 80
  dimension "d166" = 40
  dimension "d167" = 5
  dimension "d168" = 5
  constraint horizontal L1
  constraint horizontal L2
  constraint perpendicular L2 L3
  constraint horizontal L4
  constraint vertical L5
  constraint horizontal L6
  constraint vertical L7
  constraint horizontal L8
  constraint vertical L9
  constraint horizontal L10
  constraint vertical L11
  measures "d165" angle of L0 L1
  measures "d166" distance of L0.start L0.end
  measures "d167" distance of L2.end L3.end
  measures "d168" distance of L2.end L3.end
extrude "Extrude24" cut sketch "Sketch26" against normal blind 50 contours L6 L8 L9 L10 L11
sketch "Sketch27" plane through (0, 0, 5) normal (0, 0, 1) x (-1, 0, 0)
  line L0 (48.65, 1.35) -> (46.35, 1.35)
  line L1 (46.35, 1.35) -> (46.35, 3.65)
  line L2 (46.35, 3.65) -> (48.65, 3.65)
  line L3 (48.65, 3.65) -> (48.65, 1.35)
  line L4 (92, -65) -> (92, 5)
  line L5 (92, 5) -> (0, 5)
  line L6 (0, 5) -> (0, -2)
  line L7 (0, -2) -> (85.9998, -2)
  line L8 (85.9998, -2) -> (85.9998, -58)
  line L9 (85.9998, -58) -> (0, -58)
  line L10 (0, -58) -> (0, -65)
  line L11 (0, -65) -> (92, -65)
  line L12 (55.75, 3.75) -> (55.75, 1.25)
  line L13 (55.75, 1.25) -> (53.25, 1.25)
  line L14 (53.25, 1.25) -> (53.25, 3.75)
  line L15 (53.25, 3.75) -> (55.75, 3.75)
  line L16 (55.75, -63.75) -> (53.25, -63.75)
  line L17 (53.25, -63.75) -> (53.25, -61.25)
  line L18 (53.25, -61.25) -> (55.75, -61.25)
  line L19 (55.75, -61.25) -> (55.75, -63.75)
  line L20 (3.75, 3.75) -> (3.75, 1.25)
  line L21 (3.75, 1.25) -> (1.25, 1.25)
  line L22 (1.25, 1.25) -> (1.25, 3.75)
  line L23 (1.25, 3.75) -> (3.75, 3.75)
  line L24 (3.75, -63.75) -> (1.25, -63.75)
  line L25 (1.25, -63.75) -> (1.25, -61.25)
  line L26 (1.25, -61.25) -> (3.75, -61.25)
  line L27 (3.75, -61.25) -> (3.75, -63.75)
  line L28 (50, 5) -> (45, 5)
  line L29 (45, 5) -> (45, 0)
  line L30 (45, 0) -> (50, 0)
  line L31 (50, 0) -> (50, 5)
  dimension "d171" = 5
  dimension "d172" = 5
  constraint horizontal L28
  constraint vertical L29
  constraint horizontal L30
  constraint vertical L31
  constraint coincident L5 L28.start
  measures "d171" distance of L28.start L28.end
  measures "d172" distance of L28.start L30.end
extrude "Extrude25" add sketch "Sketch27" along normal blind 39.392 contours L5 L28 L29 L30 L31
sketch "Sketch28" plane through (0, 0, 5) normal (0, 0, 1) x (-1, 0, 0)
  line L0 (45, 0) -> (45, 5)
  line L1 (45, 5) -> (0, 5)
  line L2 (0, 5) -> (0, -2)
  line L3 (0, -2) -> (85.9998, -2)
  line L4 (85.9998, -2) -> (85.9998, -58)
  line L5 (85.9998, -58) -> (0, -58)
  line L6 (0, -58) -> (0, -65)
  line L7 (0, -65) -> (92, -65)
  line L8 (92, -65) -> (92, 5)
  line L9 (92, 5) -> (50, 5)
  line L10 (50, 5) -> (50, 0)
  line L11 (50, 0) -> (45, 0)
  line L12 (55.75, 3.75) -> (55.75, 1.25)
  line L13 (55.75, 1.25) -> (53.25, 1.25)
  line L14 (53.25, 1.25) -> (53.25, 3.75)
  line L15 (53.25, 3.75) -> (55.75, 3.75)
  line L16 (55.75, -63.75) -> (53.25, -63.75)
  line L17 (53.25, -63.75) -> (53.25, -61.25)
  line L18 (53.25, -61.25) -> (55.75, -61.25)
  line L19 (55.75, -61.25) -> (55.75, -63.75)
  line L20 (3.75, 3.75) -> (3.75, 1.25)
  line L21 (3.75, 1.25) -> (1.25, 1.25)
  line L22 (1.25, 1.25) -> (1.25, 3.75)
  line L23 (1.25, 3.75) -> (3.75, 3.75)
  line L24 (3.75, -63.75) -> (1.25, -63.75)
  line L25 (1.25, -63.75) -> (1.25, -61.25)
  line L26 (1.25, -61.25) -> (3.75, -61.25)
  line L27 (3.75, -61.25) -> (3.75, -63.75)
  line L28 (50, 5) -> (50, -65)
  line L29 (50, -65) -> (45, -65)
  line L30 (45, -65) -> (45, -60)
  line L31 (45, -60) -> (50, -60)
  line L32 (50, -60) -> (50, -65)
  dimension "d175" = 5
  dimension "d176" = 5
  constraint coincident L9.end L10.start
  constraint perpendicular L7 L28
  constraint horizontal L29
  constraint vertical L30
  constraint horizontal L31
  constraint vertical L32
  measures "d175" distance of L28.end L29.end
  measures "d176" distance of L28.end L31.end
extrude "Extrude26" add sketch "Sketch28" along normal blind 39.392 contours L7 L28 L29 L30 L31 L32
sketch "Sketch29" plane through (0, 0, 44.392) normal (0, 0, 1) x (-1, 0, 0)
  line L0 (50, -60) -> (45, -60)
  line L1 (45, -60) -> (45, -65)
  line L2 (45, -65) -> (50, -65)
  line L3 (50, -65) -> (50, -60)
  line L4 (50, -65) -> (50, -63.65)
  line L5 (50, -63.65) -> (48.65, -63.65)
  line L6 (48.65, -63.65) -> (46.35, -63.65)
  line L7 (46.35, -63.65) -> (46.35, -61.35)
  line L8 (46.35, -61.35) -> (48.65, -61.35)
  line L9 (48.65, -61.35) -> (48.65, -63.65)
  dimension "d179" = 1.35
  dimension "d180" = 1.35
  dimension "d181" = 2.3
  dimension "d182" = 2.3
  constraint coincident L2.end L3.start
  constraint perpendicular L2 L4
  constraint perpendicular L4 L5
  constraint horizontal L6
  constraint vertical L7
  constraint horizontal L8
  constraint vertical L9
  measures "d179" distance of L2.end L4.end
  measures "d180" distance of L4.end L5.end
  measures "d181" distance of L5.end L6.end
  measures "d182" distance of L5.end L8.end
extrude "Extrude27" add sketch "Sketch29" along normal blind 5 contours L6 L7 L8 L9
sketch "Sketch30" plane through (0, 0, 5) normal (0, 0, 1) x (-1, 0, 0)
  line L0 (3.75, -63.75) -> (1.25, -63.75)
  line L1 (1.25, -63.75) -> (1.25, -61.25)
  line L2 (1.25, -61.25) -> (3.75, -61.25)
  line L3 (3.75, -61.25) -> (3.75, -63.75)
  line L4 (3.75, 3.75) -> (3.75, 1.25)
  line L5 (3.75, 1.25) -> (1.25, 1.25)
  line L6 (1.25, 1.25) -> (1.25, 3.75)
  line L7 (1.25, 3.75) -> (3.75, 3.75)
  line L8 (55.75, -63.75) -> (53.25, -63.75)
  line L9 (53.25, -63.75) -> (53.25, -61.25)
  line L10 (53.25, -61.25) -> (55.75, -61.25)
  line L11 (55.75, -61.25) -> (55.75, -63.75)
  line L12 (55.75, 3.75) -> (55.75, 1.25)
  line L13 (55.75, 1.25) -> (53.25, 1.25)
  line L14 (53.25, 1.25) -> (53.25, 3.75)
  line L15 (53.25, 3.75) -> (55.75, 3.75)
  line L16 (45, -65) -> (45, -60)
  line L17 (45, -60) -> (50, -60)
  line L18 (50, -60) -> (50, -65)
  line L19 (50, -65) -> (92, -65)
  line L20 (92, -65) -> (92, 5)
  line L21 (92, 5) -> (50, 5)
  line L22 (50, 5) -> (50, 0)
  line L23 (50, 0) -> (45, 0)
  line L24 (45, 0) -> (45, 5)
  line L25 (45, 5) -> (0, 5)
  line L26 (0, 5) -> (0, -2)
  line L27 (0, -2) -> (85.9998, -2)
  line L28 (85.9998, -2) -> (85.9998, -58)
  line L29 (85.9998, -58) -> (0, -58)
  line L30 (0, -58) -> (0, -65)
  line L31 (0, -65) -> (45, -65)
  line L32 (45, 5) -> (5, 5)
  line L33 (5, 5) -> (10, 5)
  line L34 (10, 5) -> (10, 0)
  line L35 (10, 0) -> (5, 0)
  line L36 (5, 0) -> (5, 5)
  line L37 (45, -65) -> (5, -65)
  line L38 (5, -65) -> (10, -65)
  line L39 (10, -65) -> (10, -60)
  line L40 (10, -60) -> (5, -60)
  line L41 (5, -60) -> (5, -65)
  dimension "d185" = 40
  dimension "d186" = 5
  dimension "d187" = 5
  dimension "d188" = 40
  dimension "d189" = 5
  dimension "d190" = 5
  constraint coincident L24.end L25.start
  constraint perpendicular L24 L32
  constraint horizontal L33
  constraint vertical L34
  constraint horizontal L35
  constraint vertical L36
  constraint coincident L16.start L31.end
  constraint perpendicular L16 L37
  constraint horizontal L38
  constraint vertical L39
  constraint horizontal L40
  constraint vertical L41
  measures "d185" distance of L24.end L32.end
  measures "d186" distance of L32.end L33.end
  measures "d187" distance of L32.end L35.end
  measures "d188" distance of L16.start L37.end
  measures "d189" distance of L37.end L38.end
  measures "d190" distance of L37.end L40.end
extrude "Extrude28" add sketch "Sketch30" along normal blind 39.392 contours L31 L37 L38 L39 L40 L41 | L25 L32 L33 L34 L35 L36